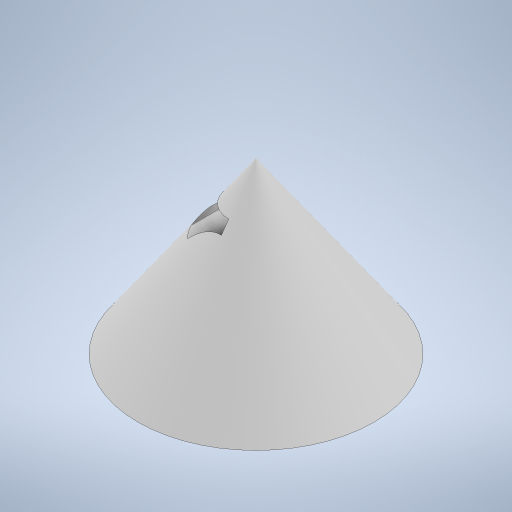
# Autodesk Inventor part: вырез
Saved by Autodesk Inventor 2023.2 (Build 272271030, 271C)
## iProperties
Created: 2023-09-16
Part Number: вырез
Material: Типовые
Document SubType Name: Modeling
Designer: User
Density: 1 g/cm^3
Appearance: По умолчанию
Author: User
Autodesk Inventor part; units mm, degrees
ref_plane "YZ Plane" through (0, 0, 0) normal (1, 0, 0) x (0, 1, 0)
ref_plane "XZ Plane" through (0, 0, 0) normal (0, 1, 0) x (-1, 0, 0)
ref_plane "XY Plane" through (0, 0, 0) normal (0, 0, 1) x (1, 0, 0)
sketch "Эскиз4" plane through (0, 0, 0) normal (1, 0, 0) x (0, 1, 0)
  line L0 (13.1772, 0) -> (-2.347, 0)
  line L1 (-2.347, 0) -> (-2.347, -10.7877)
  line L2 (-2.347, -10.7877) -> (13.1772, 0)
  point P0 (0, 0)
  constraints: 6 end point, 1 horizontal, 1 perpendicular
revolve "Вращение2" add sketch "Эскиз4" angle 360 about axis through (0, 13.1772, 0) along (0, -1, 0)
sketch "Эскиз5" plane through (0, 0, 0) normal (1, 0, 0) x (0, 1, 0)
  line L0 (13.1772, 0) -> (-2.347, -10.7877) projected
  line L1 (9.586, 3.1529) -> (6.8145, 3.1529)
  line L2 (6.8145, 3.1529) -> (6.8145, -4.4214)
  line L3 (6.8145, -4.4214) -> (9.586, -4.4214)
  line L4 (9.586, -4.4214) -> (9.586, 3.1529)
  point P0 (0, 0)
  constraints: 8 end point, 2 parallel, 1 horizontal, 1 perpendicular, 1 point on line
extrude "Выдавливание1" cut sketch "Эскиз5" against normal blind 4
